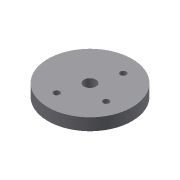
# Autodesk Inventor part: Plate
Saved by Autodesk Inventor 2022 (Build 260148000, 148)
## iProperties
Created: 2006-05-26
Part Number: Plate
Document SubType Name: Modeling
Designer: Administrator
Density: 1 g/cm^3
Material: Generic
Appearance: Default
Author: Administrator
Autodesk Inventor part; units mm, degrees
ref_plane "YZ Plane" through (0, 0, 0) normal (1, 0, 0) x (0, 1, 0)
ref_plane "XZ Plane" through (0, 0, 0) normal (0, 1, 0) x (-1, 0, 0)
ref_plane "XY Plane" through (0, 0, 0) normal (0, 0, 1) x (1, 0, 0)
sketch "Sketch1" plane through (0, 0, 0) normal (0, 0, 1) x (1, 0, 0)
  circle A0 centre (0, 0) radius 35
  dimension "d4" = 70
  constraints: 1 centre point
  measures "d4" diameter of A0
extrude "Extrusion1" add sketch "Sketch1" along normal blind 10
sketch "Sketch2" plane through (0, 0, 0) normal (0, 0, -1) x (-1, 0, 0)
  circle A0 centre (19.9717, 6.4907) radius 2.5 projected
  circle A1 centre (6.7998, -20.9228) radius 2.5 projected
  circle A2 centre (-19.9717, -6.4907) radius 2.5 projected
  circle A3 centre (-6.7998, 20.9228) radius 2.5 projected
sketch3d "3D Sketch1"
hole "Hole2" at (0, 0, 0) direction (0, 0, 1) diameter 10 end through all
hole "Hole5" at (6.7998, 20.9228, 0) at (19.9717, -6.4907, 0) at (-6.7998, -20.9228, 0) direction (0, 0, 1) diameter 5 end through all
body "Solid1"
